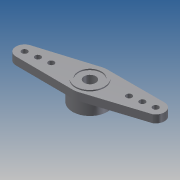
# Autodesk Inventor part: Ruderhorn
Saved by Autodesk Inventor 2012 SP2 (Build 160219200, 219)
## iProperties
Created: 2013-05-18
Part Number: Ruderhorn
Document SubType Name: Modeling
Designer: Holger
Density: 1 g/cm^3
Material: Standard
Author: Holger
Autodesk Inventor part; units mm, degrees
ref_plane "YZ Plane" through (0, 0, 0) normal (1, 0, 0) x (0, 1, 0)
ref_plane "XZ Plane" through (0, 0, 0) normal (0, 1, 0) x (-1, 0, 0)
ref_plane "XY Plane" through (0, 0, 0) normal (0, 0, 1) x (1, 0, 0)
ref_plane "Arbeitsebene7" through (0, 0, 30) normal (0, 0, 1) x (1, 0, 0)
ref_plane "Arbeitsebene1" through (8, 0, 33) normal (0, 0, 1) x (1, 0, 0)
sketch "Skizze3" plane through (8, 0, 33) normal (0, 0, 1) x (1, 0, 0)
  circle A0 centre (0, 0) radius 6.25 projected
  circle A1 centre (0, 0) radius 4.5
  point P0 (-8, 0)
  dimension "d10" = 9
  constraints: 1 centre point, 1 coincident
  measures "d10" diameter of A1
extrude "Extrusion3" add sketch "Skizze3" along normal blind 3 contours A1
sketch "Skizze4" plane through (8, 0, 36) normal (0, 0, 1) x (1, 0, 0)
  arc A0 (-15.2117, 0.0365) -> (-14.7596, -4.4148) centre (-14.7466, -2.1649) ccw
  line L0 (-0.0071, 4.5) -> (14.75, 4.5234)
  line L1 (-1.6539, 4.1851) -> (-15.593, -0.0801)
  line L2 (-14.7596, -4.4148) -> (-0.026, -4.4999)
  line L3 (15.875, 0.3269) -> (1.3639, -4.2883)
  arc A1 (-0.026, -4.4999) -> (1.3639, -4.2883) centre (0, 0) ccw
  arc A2 (-0.0071, 4.5) -> (-1.6539, 4.1851) centre (0, 0) ccw
  arc A3 (15.875, 0.3269) -> (14.7356, 4.5233) centre (14.7464, 2.2734) ccw
  point P0 (-8, 0)
  constraints: 10 point on circle, 8 end point, 4 centre point, 2 point on line, 1 tangent
extrude "Extrusion4" add sketch "Skizze4" along normal blind 2 contours L1 A2 L0 A3 L3 A1 L2 A0
ref_plane "Arbeitsebene3" through (8, 0, 38) normal (0, 0, 1) x (1, 0, 0)
sketch "Skizze5" plane through (8, 0, 38) normal (0, 0, 1) x (1, 0, 0)
  arc A0 (15.875, 0.3269) -> (14.75, 4.5234) centre (14.7464, 2.2734) ccw projected
  arc A1 (-15.593, -0.0801) -> (-14.7596, -4.4148) centre (-14.7466, -2.1649) ccw projected
  line L0 (-14.7466, -2.1649) -> (14.7464, 2.2734)
  circle A2 centre (14.7464, 2.2734) radius 0.75
  circle A3 centre (-14.7466, -2.1649) radius 0.75
  circle A4 centre (-11.7466, -1.7134) radius 0.75
  circle A5 centre (-8.7466, -1.262) radius 0.75
  circle A6 centre (11.7464, 1.8219) radius 0.75
  circle A7 centre (8.7464, 1.3705) radius 0.75
  point P0 (-8, 0)
  dimension "d21" = 3
  dimension "d22" = 3
  dimension "d23" = 3
  dimension "d24" = 3
  dimension "d25" = 1.5
  dimension "d26" = 1.5
  dimension "d27" = 1.5
  dimension "d28" = 1.5
  dimension "d29" = 1.5
  dimension "d30" = 1.5
  constraints: 6 centre point, 4 point on line, 2 coincident, 2 end point
  measures "d21" horizontal distance of A4.centre A3.centre
  measures "d22" horizontal distance of A5.centre A4.centre
  measures "d23" horizontal distance of A6.centre L0.end
  measures "d24" horizontal distance of A7.centre A6.centre
  measures "d25" diameter of A2
  measures "d26" diameter of A6
  measures "d27" diameter of A7
  measures "d28" diameter of A5
  measures "d29" diameter of A4
  measures "d30" diameter of A3
extrude "Extrusion5" cut sketch "Skizze5" against normal blind 2
ref_plane "Arbeitsebene11" through (0, 0, 31) normal (0, 0, 1) x (1, 0, 0)
ref_plane "Arbeitsebene2" through (8, 0, 38) normal (0, 0, 1) x (1, 0, 0)
sketch "Skizze12" plane through (8, 0, 38) normal (0, 0, 1) x (1, 0, 0)
  arc A0 (-0.026, -4.4999) -> (1.3639, -4.2883) centre (0, 0) ccw projected
  circle A1 centre (0, 0) radius 3
  circle A2 centre (0, 0) radius 3.75
  point P0 (-8, 0)
  dimension "d80" = 7.5
  dimension "d81" = 6
  constraints: 2 centre point, 2 coincident
  measures "d80" diameter of A2
  measures "d81" diameter of A1
extrude "Extrusion12" add sketch "Skizze12" along normal blind 0.3
ref_plane "Arbeitsebene13" through (8, 0, 38) normal (0, 0, 1) x (1, 0, 0)
sketch "Skizze13" plane through (8, 0, 38) normal (0, 0, 1) x (1, 0, 0)
  circle A0 centre (0, 0) radius 3 projected
  circle A1 centre (0, 0) radius 1.5
  point P0 (-8, 0)
  dimension "d84" = 3
  constraints: 1 centre point, 1 coincident
  measures "d84" diameter of A1
extrude "Extrusion13" cut sketch "Skizze13" against normal blind 8 contours A1
